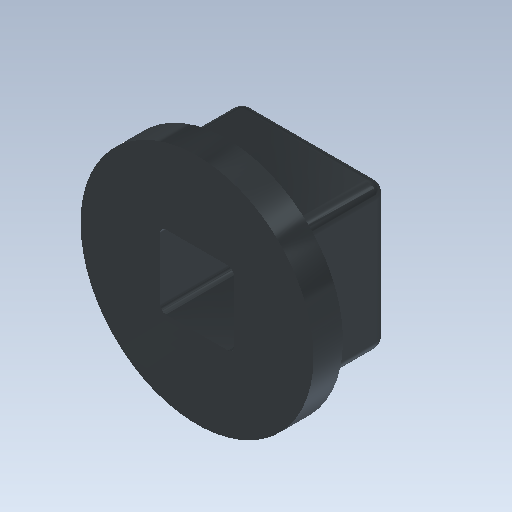
# Autodesk Inventor part: High Strength Square Gear Insert
Saved by Autodesk Inventor 2020.2 (Build 242310000, 310)
## iProperties
Created: 2012-02-22
Part Number: High Strength Square Gear Insert
Document SubType Name: Modeling
Designer: Autodesk Inc.
Density: 1.42 g/cm^3
Material: Acetal Resin, White
Catalog Web Link: http://www.vexrobotics.com/products/accessories/motion/276-2250.html#
Vendor: VEX
Mass: 0.260623 g
Surface Area: 3.24322 cm^2
Volume: 0.183538 cm^3
Appearance: Iron Gray
Category: Motion
Company: Autodesk Inc.
Author: Autodesk Inc.
Autodesk Inventor part; units mm, degrees
ref_plane "YZ Plane" through (0, 0, 0) normal (1, 0, 0) x (0, 1, 0)
ref_plane "XZ Plane" through (0, 0, 0) normal (0, 1, 0) x (-1, 0, 0)
ref_plane "XY Plane" through (0, 0, 0) normal (0, 0, 1) x (1, 0, 0)
sketch "Sketch1" plane through (0, 0, 0) normal (0, 0, 1) x (1, 0, 0)
  circle A0 centre (0, 0) radius 5.0165
  dimension "d0" = 10.033
  constraints: 1 centre point, 1 coincident
  measures "d0" diameter of A0
extrude "Extrusion1" add sketch "Sketch1" against normal blind 1.27
sketch "Sketch2" plane through (0, 0, -1.27) normal (0, 0, -1) x (-1, 0, 0)
  circle A0 centre (0, 0) radius 5.0165 projected
  line L0 (-3.1496, -3.1496) -> (3.1496, -3.1496)
  line L1 (3.1496, -3.1496) -> (3.1496, 3.1496)
  line L2 (3.1496, 3.1496) -> (-3.1496, 3.1496)
  line L3 (-3.1496, 3.1496) -> (-3.1496, -3.1496)
  point P0 (0, 3.1496)
  point P1 (-3.1496, 0)
  dimension "d3" = 6.2992
  constraints: 8 end point, 2 midpoint, 2 parallel, 2 perpendicular, 1 horizontal, 1 horizontal alignment, 1 vertical alignment
  measures "d3" distance of L1.end L2.end
extrude "Extrusion2" add sketch "Sketch2" along normal blind 3.81 contours L3 L2 L1 L0
fillet "Fillet1" radius 0.508 8 edges at (3.1496, 3.1496, -3.175) (-3.1496, 3.1496, -3.175) (-3.1496, -3.1496, -3.175) (3.1496, -3.1496, -3.175) (3.1496, 0, -5.08) (0, 3.1496, -5.08) (-3.1496, 0, -5.08) (0, -3.1496, -5.08)
sketch "Sketch4" plane through (0, 0, 0) normal (0, 0, 1) x (1, 0, 0)
  circle A0 centre (0, 0) radius 5.0165 projected
  line L0 (-1.5875, -1.5875) -> (1.5875, -1.5875)
  line L1 (1.5875, -1.5875) -> (1.5875, 1.5875)
  line L2 (1.5875, 1.5875) -> (-1.5875, 1.5875)
  line L3 (-1.5875, 1.5875) -> (-1.5875, -1.5875)
  point P0 (0, 1.5875)
  point P1 (-1.5875, 0)
  dimension "d14" = 3.175
  constraints: 8 end point, 2 midpoint, 2 parallel, 2 perpendicular, 1 horizontal, 1 horizontal alignment, 1 vertical alignment
  measures "d14" distance of L1.end L2.end
extrude "Extrusion3" cut sketch "Sketch4" against normal through all contours L3 L2 L1 L0
fillet "Fillet2" radius 0.254 4 edges at (-1.5875, 1.5875, -2.54) (1.5875, 1.5875, -2.54) (-1.5875, -1.5875, -2.54) (1.5875, -1.5875, -2.54)
sketch "Sketch5" plane through (0, 0, 0) normal (0, 0, 1) x (1, 0, 0)
  line L0 (-1.3335, 1.5875) -> (1.3335, 1.5875) projected
  circle A0 centre (0, 0) radius 5.0165 projected
  circle A1 centre (0, 0) radius 1.5875
  constraints: 1 centre point, 1 coincident, 1 tangent
surface extrude "ExtrusionSrf1" sketch "Sketch5" against normal up to surface (5.08 mm away) shown no curves A1
body "Solid1"
body "Srf1"
